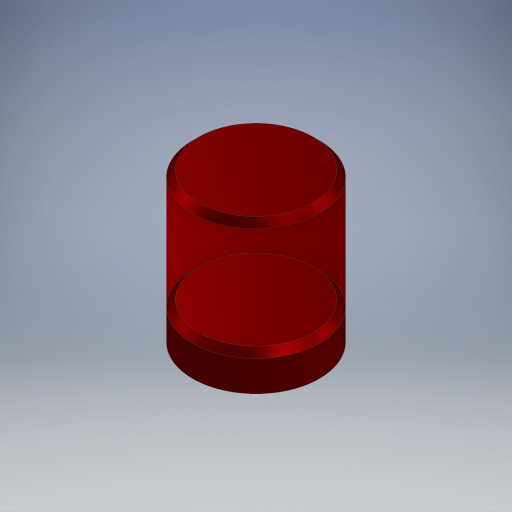
# Autodesk Inventor part: MK3-Swerve-Top-Cover
Saved by Autodesk Inventor 2024.2 (Build 282272000, 272)
## iProperties
Created: 2024-02-25
Part Number: MK3-Swerve-Top-Cover
Material: Generic
Document SubType Name: Modeling
Designer: rohan
Density: 1 g/cm^3
Appearance: Default
Author: rohan
Autodesk Inventor part; units mm, degrees
ref_plane "YZ Plane" through (0, 0, 0) normal (1, 0, 0) x (0, 1, 0)
ref_plane "XZ Plane" through (0, 0, 0) normal (0, 1, 0) x (-1, 0, 0)
ref_plane "XY Plane" through (0, 0, 0) normal (0, 0, 1) x (1, 0, 0)
sketch "Sketch1" plane through (0, 0, 0) normal (0, 1, 0) x (-1, 0, 0)
  circle A0 centre (0, 0) radius 29.21
  circle A1 centre (57.4802, -57.4802) radius 29.21
  circle A2 centre (0, 0) radius 32.385
  circle A3 centre (57.4802, -57.4802) radius 32.385
  dimension "d0" = 58.42
  dimension "d1" = 58.42
  dimension "d2" = 57.4802
  dimension "d3" = 57.4802
  dimension "d4" = 3.175
  dimension "d5" = 3.175
  constraints: 4 centre point, 1 coincident
  measures "d0" diameter of A0
  measures "d1" diameter of A1
  measures "d2" horizontal distance of A1.centre point (0, 0)
  measures "d3" horizontal distance of A1.centre point (0, 0)
  measures "d4" radial gap between concentric circles of A0 A2
  measures "d5" radial gap between concentric circles of A1 A3
extrude "Extrusion1" add sketch "Sketch1" against normal blind 14.8844
sketch "Sketch2" plane through (0, 0, 0) normal (0, 1, 0) x (1, 0, 0)
  circle A0 centre (0, 0) radius 32.385 projected
  circle A1 centre (0, 0) radius 29.21 projected
  circle A2 centre (-57.4802, 57.4802) radius 32.385 projected
  circle A3 centre (-57.4802, 57.4802) radius 29.21 projected
extrude "Extrusion2" add sketch "Sketch2" along normal blind 0.762
sketch "Sketch3" plane through (0, 0.762, 0) normal (0, 1, 0) x (1, 0, 0)
  circle A0 centre (0, 0) radius 32.385 projected
  circle A1 centre (0, 0) radius 29.21 projected
  circle A2 centre (-57.4802, 57.4802) radius 32.385 projected
  circle A3 centre (-57.4802, 57.4802) radius 29.21 projected
extrude "Extrusion3" add sketch "Sketch3" along normal blind 3.175 contours A0 | A1 | A2 | A3
chamfer "Chamfer1" distance 3.175 angle 45 2 edges at (-32.385, 3.937, 0) (-89.8652, 3.937, -57.4802)
sketch "Sketch5" plane through (0, -14.8844, 0) normal (0, -1, 0) x (1, 0, 0)
  circle A0 centre (0, 0) radius 29.21 projected
  circle A1 centre (0, 0) radius 32.385 projected
  circle A2 centre (-57.4802, -57.4802) radius 32.385 projected
  circle A3 centre (-57.4802, -57.4802) radius 29.21 projected
  circle A4 centre (-57.4802, -57.4802) radius 32.385 projected
  circle A5 centre (0, 0) radius 32.385 projected
  line L0 (-34.5805, -80.3799) -> (22.8997, -22.8997)
  line L1 (-22.8997, 22.8997) -> (-80.3799, -34.5805)
  arc A6 (-32.385, 0) -> (-32.385, 0) centre (0, 0) ccw projected
  point P0 (-45.5287, -87.5792)
  point P1 (-69.4317, -87.5792)
  point P2 (22.8997, -22.8997)
  constraints: 4 end point, 4 point on circle, 4 tangent
extrude "Extrusion5" add sketch "Sketch5" against normal blind 15.6464 contours A1 L0 A2 L1
sketch "Sketch7" plane through (-34.5805, -14.8844, -80.3799) normal (0.7071068, 0, -0.7071068) x (-0.7071068, 0, -0.7071068)
  line L0 (-68.7163, 13.6144) -> (-12.4264, 13.6144) construction
  line L1 (-12.4264, 13.6144) -> (-12.4264, 1.058) construction
  line L2 (-12.4264, 1.058) -> (-68.7163, 1.058) construction
  line L3 (-68.7163, 1.058) -> (-68.7163, 13.6144) construction
  line L4 (0, 15.6464) -> (0, 0) projected
  line L5 (-81.2893, 15.6464) -> (-81.2893, 0) projected
  line L6 (-81.2893, 15.6464) -> (0, 15.6464) projected
  line L7 (0, 0) -> (-81.2893, 0) projected
  line L8 (-61.1246, 2.1759) -> (-62.7672, 2.1759)
  line L9 (-62.7672, 2.1759) -> (-60.8523, 7.8185)
  spline S0 degree 2 poles (-60.8523, 7.8185) (-60.6991, 8.2611) (-60.3246, 9.0611) knots 0 0 0 1 1 1
  line L10 (-60.3246, 9.0611) -> (-63.78, 3.2227)
  line L11 (-63.78, 3.2227) -> (-64.6481, 3.2227)
  line L12 (-64.6481, 3.2227) -> (-64.146, 9.0611)
  spline S1 degree 2 poles (-64.146, 9.0611) (-64.3247, 8.2441) (-64.4694, 7.8185) knots 0 0 0 1 1 1
  line L13 (-64.4694, 7.8185) -> (-66.3843, 2.1759)
  line L14 (-66.3843, 2.1759) -> (-68.0269, 2.1759)
  line L15 (-68.0269, 2.1759) -> (-64.146, 13.6059)
  line L16 (-64.146, 13.6059) -> (-62.5289, 13.6059)
  line L17 (-62.5289, 13.6059) -> (-62.8779, 7.2909)
  spline S2 degree 2 poles (-62.8779, 7.2909) (-62.8864, 7.1887) (-63.014, 6.7717) knots 0 0 0 1 1 1
  spline S3 degree 2 poles (-63.014, 6.7717) (-62.9545, 6.9504) (-62.7928, 7.2909) knots 0 0 0 1 1 1
  line L18 (-62.7928, 7.2909) -> (-58.8523, 13.6059)
  line L19 (-58.8523, 13.6059) -> (-57.2437, 13.6059)
  line L20 (-57.2437, 13.6059) -> (-61.1246, 2.1759)
  line L21 (-58.0182, 2.1759) -> (-59.7289, 2.1759)
  line L22 (-59.7289, 2.1759) -> (-55.848, 13.6059)
  line L23 (-55.848, 13.6059) -> (-54.1373, 13.6059)
  line L24 (-54.1373, 13.6059) -> (-58.0182, 2.1759)
  line L25 (-50.8181, 2.1759) -> (-52.316, 2.1759)
  line L26 (-52.316, 2.1759) -> (-52.6139, 9.3675)
  spline S4 degree 2 poles (-52.6139, 9.3675) (-52.6819, 8.8484) (-52.7841, 8.542) knots 0 0 0 1 1 1
  line L27 (-52.7841, 8.542) -> (-54.9458, 2.1759)
  line L28 (-54.9458, 2.1759) -> (-56.6139, 2.1759)
  line L29 (-56.6139, 2.1759) -> (-52.733, 13.6059)
  line L30 (-52.733, 13.6059) -> (-51.2266, 13.6059)
  line L31 (-51.2266, 13.6059) -> (-50.8862, 6.5589)
  spline S5 degree 2 poles (-50.8862, 6.5589) (-50.8181, 7.0866) (-50.7159, 7.3845) knots 0 0 0 1 1 1
  line L32 (-50.7159, 7.3845) -> (-48.6053, 13.6059)
  line L33 (-48.6053, 13.6059) -> (-46.9371, 13.6059)
  line L34 (-46.9371, 13.6059) -> (-50.8181, 2.1759)
  spline S6 degree 2 poles (-43.3796, 3.078) (-43.686, 2.1759) (-44.5882, 2.1759) knots 0 0 0 1 1 1
  line L35 (-44.5882, 2.1759) -> (-48.5457, 2.1759)
  spline S7 degree 2 poles (-48.5457, 2.1759) (-49.4478, 2.1759) (-49.1414, 3.078) knots 0 0 0 1 1 1
  line L36 (-49.1414, 3.078) -> (-45.8733, 12.7037)
  spline S8 degree 2 poles (-45.8733, 12.7037) (-45.5584, 13.6059) (-44.6563, 13.6059) knots 0 0 0 1 1 1
  line L37 (-44.6563, 13.6059) -> (-40.7072, 13.6059)
  spline S9 degree 2 poles (-40.7072, 13.6059) (-39.8051, 13.6059) (-40.1115, 12.7037) knots 0 0 0 1 1 1
  line L38 (-40.1115, 12.7037) -> (-43.3796, 3.078)
  line L39 (-44.9031, 3.6397) -> (-42.0094, 12.142)
  line L40 (-42.0094, 12.142) -> (-44.3499, 12.142)
  line L41 (-44.3499, 12.142) -> (-47.2435, 3.6397)
  line L42 (-47.2435, 3.6397) -> (-44.9031, 3.6397)
  line L43 (-33.9922, 12.091) -> (-35.8731, 12.091)
  line L44 (-35.8731, 12.091) -> (-39.2434, 2.1759)
  line L45 (-39.2434, 2.1759) -> (-40.9455, 2.1759)
  line L46 (-40.9455, 2.1759) -> (-37.5753, 12.091)
  line L47 (-37.5753, 12.091) -> (-39.4562, 12.091)
  line L48 (-39.4562, 12.091) -> (-38.9455, 13.6059)
  line L49 (-38.9455, 13.6059) -> (-33.4816, 13.6059)
  line L50 (-33.4816, 13.6059) -> (-33.9922, 12.091)
  line L51 (-30.6985, 2.1759) -> (-32.3922, 2.1759)
  line L52 (-32.3922, 2.1759) -> (-32.0007, 4.3461)
  line L53 (-32.0007, 4.3461) -> (-34.1369, 4.3461)
  line L54 (-34.1369, 4.3461) -> (-35.2178, 2.1759)
  line L55 (-35.2178, 2.1759) -> (-36.9029, 2.1759)
  line L56 (-36.9029, 2.1759) -> (-36.8944, 2.2014)
  line L57 (-36.8944, 2.2014) -> (-30.8007, 13.6144)
  line L58 (-30.8007, 13.6144) -> (-29.0049, 13.6144)
  line L59 (-29.0049, 13.6144) -> (-30.6985, 2.1759)
  line L60 (-31.7369, 5.81) -> (-30.8177, 10.9675)
  line L61 (-30.8177, 10.9675) -> (-33.4135, 5.81)
  line L62 (-33.4135, 5.81) -> (-31.7369, 5.81)
  spline S10 degree 2 poles (-23.7112, 3.078) (-24.0176, 2.1759) (-24.9197, 2.1759) knots 0 0 0 1 1 1
  line L63 (-24.9197, 2.1759) -> (-28.8347, 2.1759)
  spline S11 degree 2 poles (-28.8347, 2.1759) (-29.7368, 2.1759) (-29.4304, 3.078) knots 0 0 0 1 1 1
  line L64 (-29.4304, 3.078) -> (-25.8559, 13.6059)
  line L65 (-25.8559, 13.6059) -> (-24.1452, 13.6059)
  line L66 (-24.1452, 13.6059) -> (-27.5325, 3.6397)
  line L67 (-27.5325, 3.6397) -> (-25.2346, 3.6397)
  line L68 (-25.2346, 3.6397) -> (-21.8473, 13.6059)
  line L69 (-21.8473, 13.6059) -> (-20.1367, 13.6059)
  line L70 (-20.1367, 13.6059) -> (-23.7112, 3.078)
  line L71 (-16.8004, 2.1759) -> (-18.5792, 2.1759)
  line L72 (-18.5792, 2.1759) -> (-18.6558, 7.4866)
  spline S12 degree 2 poles (-18.6558, 7.4866) (-18.4813, 8.0015) (-18.3068, 8.5164) knots 0 0 0 1 1 1
  line L73 (-18.3068, 8.5164) -> (-16.6302, 8.5164)
  line L74 (-16.6302, 8.5164) -> (-15.3961, 12.142)
  line L75 (-15.3961, 12.142) -> (-17.5494, 12.142)
  line L76 (-17.5494, 12.142) -> (-20.9367, 2.1759)
  line L77 (-20.9367, 2.1759) -> (-22.6473, 2.1759)
  line L78 (-22.6473, 2.1759) -> (-18.7664, 13.6059)
  line L79 (-18.7664, 13.6059) -> (-14.1025, 13.6059)
  spline S13 degree 2 poles (-14.1025, 13.6059) (-13.2004, 13.6059) (-13.5067, 12.7037) knots 0 0 0 1 1 1
  line L80 (-13.5067, 12.7037) -> (-15.0132, 8.2611)
  spline S14 degree 2 poles (-15.0132, 8.2611) (-15.2259, 7.6398) (-15.7791, 7.4526) knots 0 0 0 1 1 1
  spline S15 degree 2 poles (-15.7791, 7.4526) (-16.0685, 7.359) (-16.9196, 7.359) knots 0 0 0 1 1 1
  line L81 (-16.9196, 7.359) -> (-16.8004, 2.1759)
  point P0 (-81.2893, 14.8844)
  point P1 (0, 7.8232)
  point P2 (-12.4264, 7.3362)
  dimension "d59" = 81.2893
  dimension "d60" = 12.573
  dimension "d61" = 12.4263
  dimension "d62" = 2.032
  dimension "d63" = 1.058
  constraints: 2 midpoint, 2 other
  measures "d59" distance between parallel lines of L4 L5
  measures "d60" distance between parallel lines of L5 L3
  measures "d61" horizontal distance of point (0, 7.823) point (-12.426, 7.336)
  measures "d62" distance between parallel lines of L6 L0
  measures "d63" distance between parallel lines of L2 L7
extrude "Extrusion7" cut sketch "Sketch7" against normal blind 1 contours L8 L9 S0 L10 L11 L12 S1 L13 L14 L15 L16 L17 S2 S3 L18 L19 L20 | L21 L22 L23 L24 | L25 L26 S4 L27 L28 L29 L30 L31 S5 L32 L33 L34 | S6 L35 S7 L36 S8 L37 S9 L38 | L43 L44 L45 L46 L47 L48 L49 L50 | L51 L52 L53 L54 L55 L56 L57 L58 L59 | S10 L63 S11 L64 L65 L66 L67 L68 L69 L70 | L71 L72 S12 L73 L74 L75 L76 L77 L78 L79 S13 L80 S14 S15 L81
sketch "Sketch8" plane through (-22.8997, -14.8844, 22.8997) normal (-0.7071068, 0, 0.7071068) x (0.7071068, 0, 0.7071068)
  line L0 (-69.9905, 13.5882) -> (-6.6094, 13.5882) construction
  line L1 (-6.6094, 13.5882) -> (-6.6094, 1.9045) construction
  line L2 (-6.6094, 1.9045) -> (-69.9905, 1.9045) construction
  line L3 (-69.9905, 1.9045) -> (-69.9905, 13.5882) construction
  line L4 (-62.3988, 2.1497) -> (-64.0414, 2.1497)
  line L5 (-64.0414, 2.1497) -> (-62.1265, 7.7924)
  spline S0 degree 2 poles (-62.1265, 7.7924) (-61.9733, 8.2349) (-61.5988, 9.0349) knots 0 0 0 1 1 1
  line L6 (-61.5988, 9.0349) -> (-65.0542, 3.1965)
  line L7 (-65.0542, 3.1965) -> (-65.9223, 3.1965)
  line L8 (-65.9223, 3.1965) -> (-65.4202, 9.0349)
  spline S1 degree 2 poles (-65.4202, 9.0349) (-65.5989, 8.2179) (-65.7436, 7.7924) knots 0 0 0 1 1 1
  line L9 (-65.7436, 7.7924) -> (-67.6585, 2.1497)
  line L10 (-67.6585, 2.1497) -> (-69.3011, 2.1497)
  line L11 (-69.3011, 2.1497) -> (-65.4202, 13.5797)
  line L12 (-65.4202, 13.5797) -> (-63.8031, 13.5797)
  line L13 (-63.8031, 13.5797) -> (-64.1521, 7.2647)
  spline S2 degree 2 poles (-64.1521, 7.2647) (-64.1606, 7.1626) (-64.2882, 6.7455) knots 0 0 0 1 1 1
  spline S3 degree 2 poles (-64.2882, 6.7455) (-64.2287, 6.9243) (-64.067, 7.2647) knots 0 0 0 1 1 1
  line L14 (-64.067, 7.2647) -> (-60.1265, 13.5797)
  line L15 (-60.1265, 13.5797) -> (-58.5179, 13.5797)
  line L16 (-58.5179, 13.5797) -> (-62.3988, 2.1497)
  line L17 (-59.2924, 2.1497) -> (-61.0031, 2.1497)
  line L18 (-61.0031, 2.1497) -> (-57.1222, 13.5797)
  line L19 (-57.1222, 13.5797) -> (-55.4115, 13.5797)
  line L20 (-55.4115, 13.5797) -> (-59.2924, 2.1497)
  line L21 (-52.0923, 2.1497) -> (-53.5902, 2.1497)
  line L22 (-53.5902, 2.1497) -> (-53.888, 9.3413)
  spline S4 degree 2 poles (-53.888, 9.3413) (-53.9561, 8.8222) (-54.0583, 8.5158) knots 0 0 0 1 1 1
  line L23 (-54.0583, 8.5158) -> (-56.22, 2.1497)
  line L24 (-56.22, 2.1497) -> (-57.8881, 2.1497)
  line L25 (-57.8881, 2.1497) -> (-54.0072, 13.5797)
  line L26 (-54.0072, 13.5797) -> (-52.5008, 13.5797)
  line L27 (-52.5008, 13.5797) -> (-52.1604, 6.5328)
  spline S5 degree 2 poles (-52.1604, 6.5328) (-52.0923, 7.0604) (-51.9901, 7.3583) knots 0 0 0 1 1 1
  line L28 (-51.9901, 7.3583) -> (-49.8795, 13.5797)
  line L29 (-49.8795, 13.5797) -> (-48.2113, 13.5797)
  line L30 (-48.2113, 13.5797) -> (-52.0923, 2.1497)
  spline S6 degree 2 poles (-44.6538, 3.0519) (-44.9602, 2.1497) (-45.8624, 2.1497) knots 0 0 0 1 1 1
  line L31 (-45.8624, 2.1497) -> (-49.8199, 2.1497)
  spline S7 degree 2 poles (-49.8199, 2.1497) (-50.722, 2.1497) (-50.4156, 3.0519) knots 0 0 0 1 1 1
  line L32 (-50.4156, 3.0519) -> (-47.1475, 12.6776)
  spline S8 degree 2 poles (-47.1475, 12.6776) (-46.8326, 13.5797) (-45.9305, 13.5797) knots 0 0 0 1 1 1
  line L33 (-45.9305, 13.5797) -> (-41.9814, 13.5797)
  spline S9 degree 2 poles (-41.9814, 13.5797) (-41.0793, 13.5797) (-41.3857, 12.6776) knots 0 0 0 1 1 1
  line L34 (-41.3857, 12.6776) -> (-44.6538, 3.0519)
  line L35 (-46.1773, 3.6136) -> (-43.2836, 12.1159)
  line L36 (-43.2836, 12.1159) -> (-45.6241, 12.1159)
  line L37 (-45.6241, 12.1159) -> (-48.5177, 3.6136)
  line L38 (-48.5177, 3.6136) -> (-46.1773, 3.6136)
  line L39 (-35.2664, 12.0648) -> (-37.1473, 12.0648)
  line L40 (-37.1473, 12.0648) -> (-40.5176, 2.1497)
  line L41 (-40.5176, 2.1497) -> (-42.2197, 2.1497)
  line L42 (-42.2197, 2.1497) -> (-38.8495, 12.0648)
  line L43 (-38.8495, 12.0648) -> (-40.7304, 12.0648)
  line L44 (-40.7304, 12.0648) -> (-40.2197, 13.5797)
  line L45 (-40.2197, 13.5797) -> (-34.7558, 13.5797)
  line L46 (-34.7558, 13.5797) -> (-35.2664, 12.0648)
  line L47 (-31.9727, 2.1497) -> (-33.6664, 2.1497)
  line L48 (-33.6664, 2.1497) -> (-33.2749, 4.32)
  line L49 (-33.2749, 4.32) -> (-35.4111, 4.32)
  line L50 (-35.4111, 4.32) -> (-36.492, 2.1497)
  line L51 (-36.492, 2.1497) -> (-38.1771, 2.1497)
  line L52 (-38.1771, 2.1497) -> (-38.1686, 2.1752)
  line L53 (-38.1686, 2.1752) -> (-32.0749, 13.5882)
  line L54 (-32.0749, 13.5882) -> (-30.2791, 13.5882)
  line L55 (-30.2791, 13.5882) -> (-31.9727, 2.1497)
  line L56 (-33.0111, 5.7838) -> (-32.0919, 10.9414)
  line L57 (-32.0919, 10.9414) -> (-34.6877, 5.7838)
  line L58 (-34.6877, 5.7838) -> (-33.0111, 5.7838)
  spline S10 degree 2 poles (-24.9854, 3.0519) (-25.2918, 2.1497) (-26.1939, 2.1497) knots 0 0 0 1 1 1
  line L59 (-26.1939, 2.1497) -> (-30.1089, 2.1497)
  spline S11 degree 2 poles (-30.1089, 2.1497) (-31.011, 2.1497) (-30.7046, 3.0519) knots 0 0 0 1 1 1
  line L60 (-30.7046, 3.0519) -> (-27.1301, 13.5797)
  line L61 (-27.1301, 13.5797) -> (-25.4194, 13.5797)
  line L62 (-25.4194, 13.5797) -> (-28.8067, 3.6136)
  line L63 (-28.8067, 3.6136) -> (-26.5088, 3.6136)
  line L64 (-26.5088, 3.6136) -> (-23.1215, 13.5797)
  line L65 (-23.1215, 13.5797) -> (-21.4108, 13.5797)
  line L66 (-21.4108, 13.5797) -> (-24.9854, 3.0519)
  line L67 (-18.0746, 2.1497) -> (-19.8534, 2.1497)
  line L68 (-19.8534, 2.1497) -> (-19.93, 7.4604)
  spline S12 degree 2 poles (-19.93, 7.4604) (-19.7555, 7.9754) (-19.581, 8.4903) knots 0 0 0 1 1 1
  line L69 (-19.581, 8.4903) -> (-17.9044, 8.4903)
  line L70 (-17.9044, 8.4903) -> (-16.6703, 12.1159)
  line L71 (-16.6703, 12.1159) -> (-18.8236, 12.1159)
  line L72 (-18.8236, 12.1159) -> (-22.2109, 2.1497)
  line L73 (-22.2109, 2.1497) -> (-23.9215, 2.1497)
  line L74 (-23.9215, 2.1497) -> (-20.0406, 13.5797)
  line L75 (-20.0406, 13.5797) -> (-15.3767, 13.5797)
  spline S13 degree 2 poles (-15.3767, 13.5797) (-14.4745, 13.5797) (-14.7809, 12.6776) knots 0 0 0 1 1 1
  line L76 (-14.7809, 12.6776) -> (-16.2873, 8.2349)
  spline S14 degree 2 poles (-16.2873, 8.2349) (-16.5001, 7.6136) (-17.0533, 7.4264) knots 0 0 0 1 1 1
  spline S15 degree 2 poles (-17.0533, 7.4264) (-17.3427, 7.3328) (-18.1938, 7.3328) knots 0 0 0 1 1 1
  line L77 (-18.1938, 7.3328) -> (-18.0746, 2.1497)
  point P0 (0, 14.8844)
  constraints: 2 other
extrude "Extrusion8" cut sketch "Sketch8" against normal blind 1
body "Solid1"
